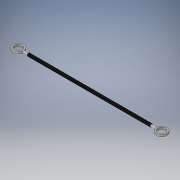
# Autodesk Inventor part: Tie Rods
Saved by Autodesk Inventor 2016 (Build 200138000, 138)
## iProperties
Created: 2015-06-02
Part Number: Tie Rods
Material: Aluminum 6061
Document SubType Name: Modeling
Designer: Dennis
Density: 2.7 g/cm^3
Appearance: Aluminum - Dark
Mass: 46.5434 g
Surface Area: 103.791 cm^2
Volume: 17.2383 cm^3
Author: Dennis
Autodesk Inventor part; units mm, degrees
ref_plane "YZ Plane" through (0, 0, 0) normal (1, 0, 0) x (0, 1, 0)
sketch "Sketch1" plane through (0, 0, 0) normal (1, 0, 0) x (0, 1, 0)
  circle A0 centre (0, 0) radius 3.7474
  constraints: 1 centre point, 1 coincident
extrude "Black Shaft" add sketch "Sketch1" along normal blind 304.8
sketch "Sketch3" plane through (304.8, 0, 0) normal (1, 0, 0) x (0, 0, -1)
  circle A0 centre (0, 0) radius 2.3813
  dimension "d2" = 4.7625
  constraints: 1 centre point, 1 coincident
  measures "d2" diameter of A0
extrude "Screwed Shaft" add sketch "Sketch3" along normal blind 12.7 and the other way blind 317.5
ref_plane "Mid Plane" through (152.4, 0, 0) normal (1, 0, 0) x (0, 0, -1)
sketch "Sketch4" plane through (0, 0, 0) normal (0, 1, 0) x (-1, 0, 0)
  circle A0 centre (25.4, 0) radius 13.0969
  line L0 (12.7, -2.3813) -> (12.7, 2.3813) construction
  circle A1 centre (25.4, 0) radius 9.525
  point P0 (0, 0)
  dimension "d7" = 26.1938
  dimension "d8" = 12.7
  dimension "d9" = 19.05
  constraints: 2 centre point, 1 coincident
  measures "d7" diameter of A0
  measures "d8" distance from line of L0 A0.centre
  measures "d9" diameter of A1
extrude "Rod End1" add sketch "Sketch4" along normal mid plane 4.7625
mirror "Rod End2" about plane through (152.4, 0, 0) normal (1, 0, 0) of "Rod End1"
ref_plane "Horizontal Midplane" through (-25.4, 0, 0) normal (0, 1, 0) x (1, 0, 0)
body "Solid1"
